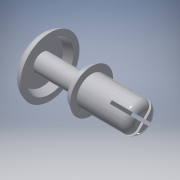
# Autodesk Inventor part: 11-6002
Saved by Autodesk Inventor 2017.1 (Build 211199000, 199)
## iProperties
Category: Quick Connect Service Pack
Company: Autodesk Inc.
Created: 2014-11-30
Part Number: 11-6002
Material: Polystyrene, High Impact
Document SubType Name: Modeling
Designer: Matrix
Density: 1.022 g/cm^3
Appearance: White
Catalog Web Link: http://matrixrobotics.com/
Vendor: Matrix
Author: Autodesk Inc.
Autodesk Inventor part; units mm, degrees
ref_plane "YZ Plane" through (0, 0, 0) normal (1, 0, 0) x (0, 1, 0)
ref_plane "XZ Plane" through (0, 0, 0) normal (0, 1, 0) x (-1, 0, 0)
ref_plane "XY Plane" through (0, 0, 0) normal (0, 0, 1) x (1, 0, 0)
sketch "Sketch1" plane through (0, 0, 0) normal (0, 1, 0) x (-1, 0, 0)
  line L0 (-1.99, -2.7996) -> (-2.9, -2.7996)
  line L1 (-2.9, -2.7996) -> (-2.3804, -1.8996)
  line L2 (-2.3804, -1.8996) -> (-1.275, -1.8996)
  line L3 (-1.275, -1.8996) -> (-1.275, -2.7996)
  line L4 (-1.275, -2.7996) -> (-1.225, -2.7996)
  line L5 (-1.225, -2.7996) -> (-1.225, 3.8354)
  line L6 (-1.225, 3.8354) -> (-2.8, 3.8354)
  line L7 (-2.8, 3.8354) -> (-3.2, 2.8354)
  line L8 (-3.2, 2.8354) -> (-4, 2.8354)
  arc A0 (-2.5786, 4.3289) -> (-4, 2.8354) centre (-2.1332, 2.4819) ccw
  arc A1 (0, 4.6354) -> (-2.5786, 4.3289) centre (0, -6.3646) ccw
  line L9 (-1.99, -8.7996) -> (-1.99, -2.7996)
  spline S0 degree 3 poles (-1.99, -8.7996) (-1.99, -8.9227) (-1.9611, -9.0675) (-1.8666, -9.2952) (-1.7841, -9.4182) (-1.6089, -9.5929) (-1.4849, -9.6753) (-1.2538, -9.7706) (-1.1056, -9.7996) (-0.9798, -9.7996) knots 0.751438 0.751438 0.751438 0.751438 0.788362 0.788362 0.82538 0.82538 0.862606 0.862606 0.900353 0.900353 0.900353 0.900353
  line L10 (0, 4.6354) -> (0, -9.7996)
  line L11 (0, -9.7996) -> (-0.9798, -9.7996)
  point P0 (0, 0)
  point P1 (0, 0)
  constraints: 24 end point, 4 point on circle, 2 centre point, 1 horizontal, 2 other
revolve "Revolution1" add sketch "Sketch1" angle 360 about axis through (0, 0, 4.6354) along (0, 0, -1)
sketch "Sketch2" plane through (0, 0, -9.7996) normal (0, 0, -1) x (-1, 0, 0)
  line L0 (0, 0.2829) -> (-1.2586, 1.5414)
  arc A0 (0.5514, 0.8343) -> (-0.5514, 0.8343) centre (0, 0) ccw
  line L1 (1.2586, 1.5414) -> (0, 0.2829)
  line L2 (0, -0.2829) -> (1.2585, -1.5414)
  arc A1 (-0.5514, -0.8343) -> (0.5514, -0.8343) centre (0, 0) ccw
  line L3 (-1.2586, -1.5414) -> (0, -0.2829)
  line L4 (0.2829, 0) -> (1.5414, 1.2586)
  arc A2 (0.8343, -0.5514) -> (0.8343, 0.5514) centre (0, 0) ccw
  line L5 (1.5414, -1.2585) -> (0.2829, 0)
  arc A3 (-0.8343, 0.5514) -> (-0.8343, -0.5514) centre (0, 0) ccw
  line L6 (-0.2829, 0) -> (-1.5414, -1.2585)
  line L7 (-1.5414, 1.2586) -> (-0.2829, 0)
  arc A4 (-1.2657, -1.5485) -> (1.2657, -1.5485) centre (0, 0) ccw
  circle A5 centre (0, 0) radius 1.99 projected
  point P0 (0, 0)
  point P1 (0, 0)
  point P2 (-1.99, 0)
  constraints: 16 end point, 10 point on circle, 8 point on line, 5 centre point, 9 other
extrude "Extrusion1" cut sketch "Sketch2" against normal blind 3 contours L1 A5 L4 L5 L2 L3 L6 L7 L0
body "Solid1"
